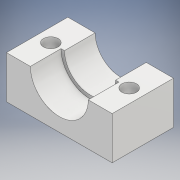
# Autodesk Inventor part: Colimador inferior
Saved by Autodesk Inventor 2019.4 (Build 234330000, 330)
## iProperties
Created: 2018-03-06
Part Number: Colimador inferior
Material: Generic
Document SubType Name: Modeling
Designer: Hogar
Density: 1 g/cm^3
Appearance: White
Author: Hogar
Autodesk Inventor part; units mm, degrees
ref_plane "YZ Plane" through (0, 0, 0) normal (1, 0, 0) x (0, 1, 0)
ref_plane "XZ Plane" through (0, 0, 0) normal (0, 1, 0) x (-1, 0, 0)
ref_plane "XY Plane" through (0, 0, 0) normal (0, 0, 1) x (1, 0, 0)
sketch "Sketch1" plane through (0, 0, 0) normal (0, 0, 1) x (1, 0, 0)
  line L0 (-15.5, -9) -> (15.5, -9)
  line L1 (15.5, -9) -> (15.5, 9)
  line L2 (15.5, 9) -> (-15.5, 9)
  line L3 (-15.5, 9) -> (-15.5, -9)
  line L4 (-15.5, -9) -> (15.5, 9) construction
  line L5 (15.5, -9) -> (-15.5, 9) construction
  point P0 (0, 0)
  dimension "d0" = 31
  dimension "d1" = 18
  constraints: 12 end point, 2 midpoint, 2 parallel, 1 horizontal, 1 perpendicular
  measures "d0" distance of L2.end L1.end
  measures "d1" distance of L1.end L0.end
extrude "Extrusion1" add sketch "Sketch1" along normal blind 12.5
sketch "Sketch4" plane through (-15.5, -9, 0) normal (0, -1, 0) x (1, 0, 0)
  line L0 (0, 12.5) -> (31, 12.5) projected
  circle A0 centre (15.5, 12.5) radius 7.5
  point P0 (15.5, 0)
  dimension "d24" = 15
  constraints: 1 centre point, 1 midpoint
  measures "d24" diameter of A0
extrude "Extrusion4" cut sketch "Sketch4" against normal through all
sketch "Sketch5" plane through (0, 0, 12.5) normal (0, 0, 1) x (1, 0, 0)
  line L0 (-15.5, -9) -> (-7.5, -9) projected
  line L1 (7.5, -9) -> (15.5, -9) projected
  point P0 (0, 0)
  point P1 (-11.5, 0)
  point P2 (11.5, 0)
  dimension "d86" = 11.5
  dimension "d87" = 11.5
  dimension "d88" = 9
  dimension "d89" = 9
  measures "d86" distance of point (0, 0) point (-11.5, 0)
  measures "d87" distance of point (11.5, 0) point (0, 0)
  measures "d88" distance from line of point (-11.5, 0) L0
  measures "d89" distance from line of L1 point (11.5, 0)
sketch "Sketch8" plane through (-15.5, 9, 0) normal (0, 1, 0) x (1, 0, 0)
  circle A0 centre (6.1, -9.5) radius 1.5
  line L0 (8, -12.5) -> (0, -12.5) projected
  line L1 (0, 0) -> (0, -12.5) projected
  point P0 (15.5, 0)
  dimension "d57" = 3
  dimension "d59" = 3
  dimension "d61" = 6.1
  constraints: 1 centre point
  measures "d57" diameter of A0
  measures "d59" distance from line of L0 A0.centre
  measures "d61" distance from line of L1 A0.centre
hole "Hole1" at (-11.5, 0, 12.5) at (11.5, 0, 12.5) direction (0, 0, -1) diameter 4.3 end through all clearance for "Flat Head Machine Screw" size "M4" standard "Ansi Metric M Profile"
extrude "Extrusion11" cut sketch "Sketch8" against normal blind 5.2
sketch "Sketch13" plane through (-15.5, -9, 0) normal (0, -1, 0) x (1, 0, 0)
  arc A0 (8, 12.5) -> (23, 12.5) centre (15.5, 12.5) ccw projected
  circle A1 centre (15.5, 12.5) radius 8.5
  point P0 (15.5, 0)
  dimension "d99" = 17
  constraints: 1 centre point, 1 coincident
  measures "d99" diameter of A1
extrude "Extrusion12" cut sketch "Sketch13" against normal blind 9
equation "\"d87\" = d86"
equation "\"d89\" = d88"
body "Solid1"
